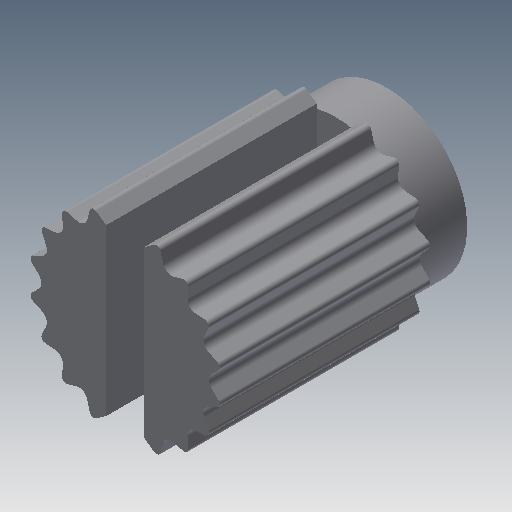
# Autodesk Inventor part: Part5_panel pot
Saved by Autodesk Inventor 2020 (Build 240168000, 168)
## iProperties
Created: 2016-08-22
Part Number: Part5_panel pot
Material: Generic
Document SubType Name: Modeling
Designer: Tom
Density: 1 g/cm^3
Appearance: Default
Author: Tom
Autodesk Inventor part; units mm, degrees
ref_plane "YZ Plane" through (0, 0, 0) normal (1, 0, 0) x (0, 1, 0)
ref_plane "XZ Plane" through (0, 0, 0) normal (0, 1, 0) x (-1, 0, 0)
ref_plane "XY Plane" through (0, 0, 0) normal (0, 0, 1) x (1, 0, 0)
sketch "Sketch1" plane through (0, 0, 0) normal (0, 0, 1) x (1, 0, 0)
  circle A0 centre (0, 0) radius 3.0315
  dimension "d0" = 6.063
  constraints: 1 centre point, 1 coincident
  measures "d0" diameter of A0
extrude "Extrusion1" add sketch "Sketch1" along normal blind 7.2644
sketch "Sketch2" plane through (0, 0, 7.2644) normal (0, 0, 1) x (1, 0, 0)
  circle A0 centre (0, 0) radius 3.0315 projected
  line L0 (-0.5842, -3.6567) -> (0.5842, -3.6567)
  line L1 (0.5842, -3.6567) -> (0.5842, 3.7865)
  line L2 (0.5842, 3.7865) -> (-0.5842, 3.7865)
  line L3 (-0.5842, 3.7865) -> (-0.5842, -3.6567)
  dimension "d3" = 1.1684
  dimension "d4" = 0.5842
  constraints: 8 end point, 2 parallel, 1 horizontal, 1 perpendicular
  measures "d3" distance of L1.end L2.end
  measures "d4" horizontal distance of L1.end A0.centre
extrude "Extrusion2" cut sketch "Sketch2" against normal through all contours L1 A0 L3 | A0 L3 L2 L1 | L1 L0 L3 A0
sketch "Sketch8" plane through (0, 0, 7.2644) normal (0, 0, 1) x (1, 0, 0)
  line L0 (0.5842, 2.9747) -> (0.5842, -2.9747) projected
  arc A0 (0.5842, -2.9747) -> (0.5842, 2.9747) centre (0, 0) ccw projected
  line L1 (0, 0) -> (3.0881, 0) construction
  line L2 (2.4806, 0) -> (2.9886, -0.508)
  line L3 (2.4806, 0) -> (2.9886, 0.508)
  dimension "d32" = 0.508
  dimension "d33" = 90
  dimension "d34" = 45
  dimension "d35" = 1.016
  constraints: 6 end point, 2 perpendicular, 2 point on circle, 1 point on line
  measures "d32" horizontal distance of L3.end L2.start
  measures "d33" angle of L3 L2
  measures "d34" angle of L1 L3
  measures "d35" distance of L3.end L2.end
extrude "Extrusion6" cut sketch "Sketch8" against normal through all contours A0 L2 L3
fillet "Fillet1" radius 0.254 1 edges at (2.4806, 0, 3.6322)
pattern_circular "Circular Pattern1" count 18 over 360 about axis through (0, 0, 0) along (0, 0, 1) of "Extrusion6"
sketch "Sketch9" plane through (0, 0, 0) normal (0, 0, -1) x (-1, 0, 0)
  arc A0 (1.0544, 2.8422) -> (1.0193, 2.855) centre (0, 0) ccw projected
  circle A1 centre (0, 0) radius 2.4806
  constraints: 1 centre point, 1 coincident
extrude "Extrusion7" add sketch "Sketch9" along normal blind 0.8128
fillet "Fillet2" radius 0.127 16 edges at (1.9629, 2.3102, 3.6322) (1.9343, 2.3342, 3.6322) (1.0544, 2.8422, 3.6322) (1.0193, 2.855, 3.6322) (2.6346, 1.4995, 3.6322) (2.616, 1.5319, 3.6322) (2.9821, 0.5448, 3.6322) (2.9886, 0.508, 3.6322) (2.9886, -0.508, 3.6322) (2.9821, -0.5448, 3.6322) (2.6346, -1.4995, 3.6322) (2.616, -1.5319, 3.6322) (1.9629, -2.3102, 3.6322) (1.9343, -2.3342, 3.6322) (1.0544, -2.8422, 3.6322) (1.0193, -2.855, 3.6322)
fillet "Fillet3" radius 0.127 16 edges at (-1.0544, -2.8422, 3.6322) (-1.0193, -2.855, 3.6322) (-1.9343, -2.3342, 3.6322) (-1.9629, -2.3102, 3.6322) (-2.616, -1.5319, 3.6322) (-2.6346, -1.4995, 3.6322) (-2.9821, -0.5448, 3.6322) (-2.9886, -0.508, 3.6322) (-2.9821, 0.5448, 3.6322) (-2.9886, 0.508, 3.6322) (-2.6346, 1.4995, 3.6322) (-2.616, 1.5319, 3.6322) (-1.9629, 2.3102, 3.6322) (-1.9343, 2.3342, 3.6322) (-1.0544, 2.8422, 3.6322) (-1.0193, 2.855, 3.6322)
move faces "Move Face1" translate (0, 0, 0.762) faces at (-0.1947, 0.8036, 0)
sketch "Sketch10" plane through (0, 0, 0) normal (0, 0, 1) x (1, 0, 0)
  point P0 (0, 0)
move faces "Move Face2" translate (0, 0, 0.762) faces at (-2.287, 1.2804, 0) (-2.587, 0.4209, 0) (-2.575, -0.4892, 0) (-2.2523, -1.3404, 0) (-1.6581, -2.0299, 0) (-0.7642, -2.5548, 0) (0.7642, -2.5548, 0) (1.6581, -2.0299, 0) (2.287, -1.2804, 0) (2.5474, 0.5814, 0) (2.2523, 1.3404, 0) (1.7112, 1.9854, 0) (0.7642, 2.5548, 0) (-0.7642, 2.5548, 0) (-1.7112, 1.9854, 0)
fillet "Fillet4" radius 0.254 13 edges at (2.331, 0.8484, 4.0132) (1.9003, 1.5945, 4.0132) (1.2403, 2.1483, 4.0132) (2.331, -0.8484, 4.0132) (1.9003, -1.5945, 4.0132) (1.2403, -2.1483, 4.0132) (-1.2403, -2.1483, 4.0132) (-1.9003, -1.5945, 4.0132) (-2.331, -0.8484, 4.0132) (-2.4806, 0, 4.0132) (-2.331, 0.8484, 4.0132) (-1.9003, 1.5945, 4.0132) (-1.2403, 2.1483, 4.0132)
equation "\"d4\" = 0.5 * d3"
equation "\"d34\" = 0.5 * d33"
body "Solid1"
